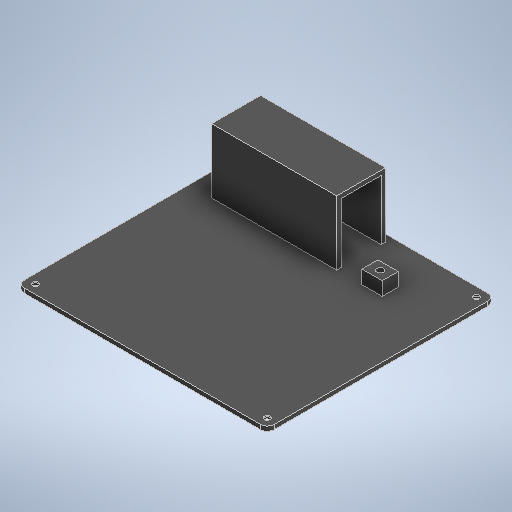
# Autodesk Inventor part: podstawa
Saved by Autodesk Inventor 2025 (Build 290162000, 162)
## iProperties
Created: 2026-04-02
Part Number: podstawa
Material: Ogólny
Document SubType Name: Modeling
Designer: zzapa
Density: 1 g/cm^3
Appearance: Ogólny
Author: zzapa
Autodesk Inventor part; units mm, degrees
ref_plane "YZ Plane" through (0, 0, 0) normal (1, 0, 0) x (0, 1, 0)
ref_plane "XZ Plane" through (0, 0, 0) normal (0, 1, 0) x (-1, 0, 0)
ref_plane "XY Plane" through (0, 0, 0) normal (0, 0, 1) x (1, 0, 0)
sketch "Szkic1" plane through (0, 0, 0) normal (0, 1, 0) x (-1, 0, 0)
  line L0 (110, 0) -> (0, 0)
  line L1 (0, 0) -> (0, -100)
  line L2 (0, -100) -> (110, -100)
  line L3 (110, -100) -> (110, 0)
  dimension "d0" = 100
  dimension "d1" = 110
  constraints: 8 end point, 2 parallel, 1 coincident, 1 horizontal, 1 perpendicular
  measures "d0" distance of L2.end L0.start
  measures "d1" distance of L1.end L2.end
extrude "Gabaryt" add sketch "Szkic1" along normal blind 2
sketch "Szkic2" plane through (0, 0, 0) normal (0, 1, 0) x (1, 0, 0)
  line L0 (0, 0) -> (0, 100) projected
  line L1 (-110, 0) -> (0, 0) projected
  line L2 (-110, 100) -> (-110, 0) projected
  line L3 (0, 100) -> (-110, 100) projected
  line L4 (-110, 50) -> (0, 50)
  line L5 (-55, 100) -> (-55, 0)
  point P0 (-4, 4)
  point P1 (-106, 4)
  point P2 (-4, 96)
  point P3 (-106, 96)
  dimension "d4" = 4
  dimension "d5" = 4
  constraints: 4 end point, 4 midpoint, 3 symmetric about line
  measures "d4" distance from line of point (-4, 4) L0
  measures "d5" distance from line of L1 point (-4, 4)
hole "Otwory montażowe" at (-4, 0, -4) at (-106, 0, -4) at (-106, 0, -96) at (-4, 0, -96) direction (0, 1, 0) diameter 2.6 end through all counterbore diameter 4.5 counterbore depth 1.5
fillet "Zaokrąglenie1" radius 3 4 edges at (0, 1, 0) (-110, 1, 0) (-110, 1, -100) (0, 1, -100)
ref_plane "Płaszczyzna konstrukcyjna2" through (-100, 0, -97) normal (-1, 0, 0) x (0, 0, 1)
sketch "Szkic4" plane through (-100, 0, -97) normal (-1, 0, 0) x (0, 0, 1)
  line L0 (0, 2) -> (94, 2) projected
  line L1 (0, 28.3) -> (2, 28.3)
  line L2 (2, 28.3) -> (2, 2)
  line L3 (2, 2) -> (0, 2)
  line L4 (0, 2) -> (0, 28.3)
  line L5 (19.5, 28.3) -> (21.5, 28.3)
  line L6 (21.5, 28.3) -> (21.5, 2)
  line L7 (21.5, 2) -> (19.5, 2)
  line L8 (19.5, 2) -> (19.5, 28.3)
  line L9 (0, 30.3) -> (21.5, 30.3)
  line L10 (21.5, 30.3) -> (21.5, 28.3)
  line L11 (21.5, 28.3) -> (0, 28.3)
  line L12 (0, 28.3) -> (0, 30.3)
  line L13 (-3, 2) -> (-3, 0) projected
  point P0 (97, 0)
  point P1 (2, 2)
  point P2 (2, 28.3)
  point P3 (19.5, 2)
  point P4 (21.5, 2)
  dimension "d20" = 2
  dimension "d21" = 2
  dimension "d22" = 2
  dimension "d23" = 17.5
  dimension "d24" = 26.3
  dimension "d25" = 3
  constraints: 24 end point, 6 collinear, 6 parallel, 3 horizontal, 3 perpendicular
  measures "d20" distance between parallel lines of L4 L2
  measures "d21" distance between parallel lines of L11 L9
  measures "d22" distance between parallel lines of L8 L6
  measures "d23" distance between parallel lines of L8 L2
  measures "d24" distance between parallel lines of L0 L11
  measures "d25" distance between parallel lines of L13 L4
extrude "Wyciągnięcie proste3" add sketch "Szkic4" against normal blind 55 contours L4 L1 L2 L0 | L12 L9 L10 L5 L11 L1 | L8 L5 L6 L0
sketch "Szkic5" plane through (0, 2, 0) normal (0, 1, 0) x (1, 0, 0)
  line L0 (-33.9, 82.5) -> (-25, 82.5)
  line L1 (-25, 82.5) -> (-25, 75.5)
  line L2 (-25, 75.5) -> (-33.9, 75.5)
  line L3 (-33.9, 75.5) -> (-33.9, 82.5)
  line L4 (-100, 75.5) -> (-45, 75.5) projected
  line L5 (-110, 97) -> (-110, 3) projected
  line L6 (0, 3) -> (0, 97) projected
  point P0 (0, 0)
  point P1 (-29.45, 82.5)
  dimension "d28" = 7
  dimension "d29" = 8.9
  dimension "d34" = 25
  constraints: 8 end point, 2 parallel, 1 collinear, 1 horizontal, 1 midpoint, 1 perpendicular
  measures "d28" distance of L0.end L1.end
  measures "d29" distance of L0.start L0.end
  measures "d34" distance between parallel lines of L6 L1
extrude "Wyciągnięcie proste4" add sketch "Szkic5" along normal blind 6
sketch "Szkic6" plane through (0, 8, 0) normal (0, 1, 0) x (1, 0, 0)
  line L0 (-25, 82.5) -> (-33.9, 82.5) projected
  line L1 (-33.9, 82.5) -> (-33.9, 75.5) projected
  line L2 (-33.9, 75.5) -> (-25, 75.5) projected
  line L3 (-25, 75.5) -> (-25, 82.5) projected
  line L4 (-33.9, 75.5) -> (-33.9, 82.5) projected
  line L5 (-33.9, 79) -> (-25, 79)
  line L6 (-29.45, 82.5) -> (-29.45, 75.5)
  point P0 (0, 0)
  point P1 (-29.45, 79)
  constraints: 6 midpoint, 4 end point
hole "Otwór2" at (-29.45, 8, -79) direction (0, -1, 0) diameter 2.9 depth 7
equation "\"d0\" = podstawa_a"
equation "\"d1\" = podstawa_b"
equation "\"d2\" = podstawa_wys"
equation "\"d4\" = podstawa_otwory_montazowe_poz_x"
equation "\"d5\" = podstawa_otwory_montazowe_poz_y"
equation "\"d6\" = gniazdo_M2_D2"
equation "\"d8\" = gniazdo_M2_D1"
equation "\"d9\" = gniazdo_M2_glebokosc"
equation "\"d13\" = podstawa_zaokraglenie"
equation "\"d20\" = obudowa_uchwyt_grubosc"
equation "\"d21\" = d20"
equation "\"d22\" = d20"
equation "\"d23\" = obudowa_uchwyt_szerokosc_wew"
equation "\"d24\" = obudowa_uchwyt_wysokosc_wew"
equation "\"d25\" = obudowa_uchwyt_poz_z"
equation "\"d26\" = obudowa_uchwyt_kolnierz_wys"
equation "\"d28\" = podstawa_mocowanie_DC_a"
equation "\"d29\" = podstawa_mocowanie_DC_b"
equation "\"d34\" = obudowa_gniazdo_poz"
equation "\"d32\" = podstawa_mocowanie_DC_wys"
equation "\"d35\" = insert_D"
equation "\"d37\" = gniazdo_M2_D1"
equation "\"d38\" = gniazdo_M2_glebokosc"
equation "\"d40\" = insert_glebokosc"
equation "\"podstawa_a\" = 100"
equation "\"podstawa_b\" = 110"
equation "\"podstawa_wys\" = 2"
equation "\"podstawa_otwory_montazowe_poz_y\" = 4"
equation "\"podstawa_otwory_montazowe_poz_x\" = 4"
equation "\"gniazdo_M2_D1\" = 4.5"
equation "\"gniazdo_M2_glebokosc\" = 1.5"
equation "\"gniazdo_M2_D2\" = 2.6"
equation "\"obudowa_wys\" = 45"
equation "\"obudowa_grubosc\" = 2"
equation "\"obudowa_prowadnica_odsuniecie\" = 2"
equation "\"obudowa_prowadnica_grubosc\" = 2"
equation "\"obudowa_kontrolki_a\" = 38"
equation "\"obudowa_prowadnica_wys\" = 19"
equation "\"obudowa_otwory_montazowe_poz_y\" = 4"
equation "\"obudowa_otwory_montazowe_poz_x\" = 4"
equation "\"obudowa_otwory_montazowe_material_y\" = 8"
equation "\"obudowa_otwory_montazowe_material_x\" = 8"
equation "\"insert_D\" = 2.9"
equation "\"insert_glebokosc\" = 7"
equation "\"obudowa_zaokraglenie\" = 3"
equation "\"podstawa_zaokraglenie\" = 3"
equation "\"obudowa_otwory_io_wys\" = 15"
equation "\"obudowa_otwory_io_D\" = 15"
equation "\"obudowa_otwory_io1_poz\" = 55"
equation "\"obudowa_otwory_io1_wys\" = 25"
equation "\"obudowa_otwory_io1_D\" = 12"
equation "\"obudowa_otwory_io2_poz\" = 38"
equation "\"obudowa_otwory_io2_wys\" = 25"
equation "\"obudowa_otwory_io2_D\" = 12"
equation "\"obudowa_otwory_pot_D\" = 7.2"
equation "\"input_b\" = 14.4"
equation "\"input_wys\" = 10.9"
equation "\"input_a\" = 8.9"
equation "\"obudowa_MTS_otwor_D\" = 6.2"
equation "\"obudowa_pot_poz_y\" = 15"
equation "\"obudowa_s_poz_x\" = 78"
equation "\"obudowa_s_D\" = 6.2"
equation "\"obudowa_s_poz_y\" = 15"
equation "\"obudowa_s_rozstaw_y\" = 16"
equation "\"pcb_rozstaw_x\" = 92"
equation "\"pcb_rozstaw_y\" = 58"
equation "\"obudowa_pcb_grubosc_scianki\" = 6"
equation "\"pcb_grubosc_scianki\" = 6"
equation "\"pcb_poz_y\" = 29"
equation "\"pcb_wys_bloku\" = 35"
equation "\"obudowa_footswitch_poz_y\" = 68"
equation "\"obudowa_footswitch_poz_x\" = 35"
equation "\"obudowa_footswitch_D\" = 12.3"
equation "\"obudowa_led_indicator_D\" = 3.5"
equation "\"obudowa_led_indicator_poz_x\" = 55"
equation "\"obudowa_podkladka_otwory\" = 4"
equation "\"podstawa_uchwyt_grubosc\" = 3"
equation "\"podstawa_uchwyt_wysokosc\" = 15"
equation "\"obudowa_uchwyt_grubosc\" = 2"
equation "\"pbudowa_uchwyt_podciecie_wys\" = 1.5"
equation "\"obudowa_uchwyt_wysokosc_wew\" = 26.3"
equation "\"obudowa_uchwyt_szerokosc_wew\" = 17.5"
equation "\"obudowa_gniazdo_poz\" = 25"
equation "\"obudowa_uchwyt_kolnierz_wys\" = 55"
equation "\"obudowa_uchwyt_poz_y\" = 2"
equation "\"obudowa_uchwyt_poz_z\" = 3"
equation "\"obudowa_podciecie_inout_wys\" = 6"
equation "\"obudowa_podciecie_logo_wys\" = 34"
equation "\"obudowa_podciecie_logo_szerokosc\" = 25"
equation "\"obudowa_pot_pozycjonowanie_wys\" = 13"
equation "\"obudowa_pot_pozycjonowanie_szerokosc\" = 2.8"
equation "\"obudowa_pot_pozycjonowanie_glebokosc\" = 1.4"
equation "\"obudowa_led_mocowanie_wys\" = 6"
equation "\"obudowa_led_mocowanie_poz\" = 46"
equation "\"obudowa_led_mocowanie_D\" = 5.5"
equation "\"obudowa_led_mocowanie_grubosc\" = 8"
equation "\"holder_led_grubosc\" = 2.5"
equation "\"holder_led_dlugosc\" = 28"
equation "\"holder_led_uchwyt_D\" = 5"
equation "\"holder_led_uchwyt_wysokosc\" = 5"
equation "\"holder_led_uchwyt_szerokosc\" = 8"
equation "\"holder_gniazdo_b\" = 5"
equation "\"holder_gniazdo_grubosc\" = 2.5"
equation "\"holder_gniazdo_a\" = 28"
equation "\"podstawa_mocowanie_DC_a\" = 7"
equation "\"podstawa_mocowanie_DC_b\" = 8.9"
equation "\"podstawa_mocowanie_DC_wys\" = 6"
equation "\"holder_gniazdo_odleglosc_miedzy_ramionami\" = 9.2"
equation "\"holder_gniazdo_grubosc_ramion\" = 1.5"
equation "\"holder_gniazdo_wys\" = 8"
equation "\"holder_gniazdo_uchwyt_poz\" = 5"
